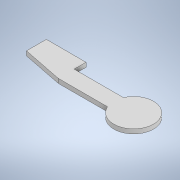
# Autodesk Inventor part: PINZA_I
Saved by Autodesk Inventor 2022 (Build 260153000, 153)
## iProperties
Created: 2022-11-02
Part Number: PINZA_I
Material: Genérico
Document SubType Name: Modeling
Designer: Usuario
Density: 1 g/cm^3
Appearance: Valor por defecto
Author: Usuario
Autodesk Inventor part; units mm, degrees
ref_plane "YZ Plane" through (0, 0, 0) normal (1, 0, 0) x (0, 1, 0)
ref_plane "XZ Plane" through (0, 0, 0) normal (0, 1, 0) x (-1, 0, 0)
ref_plane "XY Plane" through (0, 0, 0) normal (0, 0, 1) x (1, 0, 0)
sketch "Boceto1" plane through (0, 0, 0) normal (0, 1, 0) x (-1, 0, 0)
  line L0 (50, 10) -> (-50, 10)
  line L1 (-50, 10) -> (-50, -10)
  line L2 (-50, -10) -> (50, -10)
  line L3 (50, -10) -> (50, 10)
  line L4 (50, 10) -> (-50, -10) construction
  line L5 (-50, 10) -> (50, -10) construction
  line L6 (-50, -10) -> (-20, -10)
  line L7 (0, 0) -> (50, 0)
  line L8 (0, 0) -> (0, 10)
  dimension "d0" = 100
  dimension "d1" = 20
  dimension "d2" = 30
  constraints: 18 end point, 4 midpoint, 2 parallel, 1 horizontal, 1 perpendicular, 1 point on line
  measures "d0" distance of L2.end L1.end
  measures "d1" distance of L1.end L0.end
  measures "d2" distance of L1.end L6.end
extrude "Extrusión1" add sketch "Boceto1" along normal blind 5.5 contours L3 L7 L8 L0
extrude "Extrusión2" add sketch "Boceto1" along normal blind 5.5 contours L8 L7 L3 L2 L1 L0
sketch "Boceto5" plane through (0, 5.5, 0) normal (0, 1, 0) x (1, 0, 0)
  line L0 (50, 10) -> (-50, 10) projected
  line L1 (20, 0) -> (50, 0)
  circle A0 centre (35, 0) radius 25
  line L2 (35, 25) -> (35, 20)
  line L3 (35, 20) -> (50, 20)
  line L4 (35, 20) -> (20, 20)
  line L5 (35, 0) -> (50, 0)
  point P0 (0, 0)
  point P1 (20, 10)
  dimension "d27" = 50
  constraints: 10 end point, 3 point on circle, 1 centre point, 1 collinear, 1 midpoint, 1 perpendicular, 1 point on line, 1 vertical
  measures "d27" diameter of A0
extrude "Extrusión8" add sketch "Boceto5" against normal blind 5.5
sketch "Boceto6" plane through (0, 5.5, 0) normal (0, 1, 0) x (1, 0, 0)
  line L0 (12.0871, 10) -> (-50, 10) projected
  line L1 (-50, 10) -> (-50, -10) projected
  line L2 (-50, -10) -> (12.0871, -10) projected
  arc A0 (12.0871, -10) -> (12.0871, 10) centre (35, 0) ccw projected
  line L3 (-50, 10) -> (-50, -10) projected
  line L4 (-50, 0) -> (-100, 0)
  line L5 (-100, 0) -> (-50, -10)
  line L6 (-100, 0) -> (-100, 50)
  line L7 (-100, 50) -> (-50, 50)
  line L8 (-50, 50) -> (-50, 0)
  line L9 (-100, 25) -> (-50, 25)
  point P0 (0, 0)
  dimension "d33" = 50
  dimension "d34" = 50
  constraints: 12 end point, 3 midpoint, 1 collinear, 1 horizontal, 1 perpendicular, 1 vertical
  measures "d33" distance of L4.start L4.end
  measures "d34" distance of L4.end L6.end
extrude "Extrusión9" add sketch "Boceto6" against normal blind 5.5 contours L1 L4 L6 L9 L8 | L1 L5 L4
